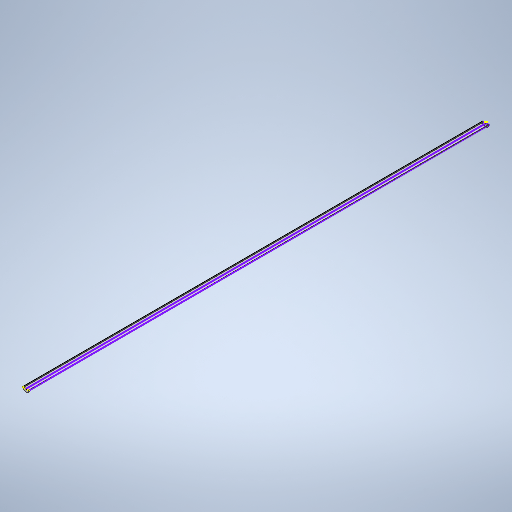
# Autodesk Inventor part: Tubo
Saved by Autodesk Inventor 2025.3 (Build 293356000, 356)
## iProperties
Created: 2025-11-02
Part Number: Tubo
Material: Genérico
Document SubType Name: Modeling
Designer: PAVILION
Density: 1 g/cm^3
Appearance: Valor por defecto
Author: PAVILION
Autodesk Inventor part; units mm, degrees
ref_plane "YZ Plane" through (0, 0, 0) normal (1, 0, 0) x (0, 1, 0)
ref_plane "XZ Plane" through (0, 0, 0) normal (0, 1, 0) x (-1, 0, 0)
ref_plane "XY Plane" through (0, 0, 0) normal (0, 0, 1) x (1, 0, 0)
sketch "Boceto1" plane through (0, 0, 0) normal (0, 0, 1) x (1, 0, 0)
  circle A0 centre (0, 0) radius 38.1
  circle A1 centre (0, 0) radius 34
  dimension "d0" = 76.2
  dimension "d1" = 68
  constraints: 2 centre point, 2 coincident
  measures "d0" diameter of A0
  measures "d1" diameter of A1
extrude "Extrusión1" add sketch "Boceto1" along normal blind 6100
sketch "Boceto2" plane through (0, 0, 6100) normal (0, 0, 1) x (1, 0, 0)
  circle A0 centre (0, 0) radius 39.5
  circle A1 centre (0, 0) radius 34 projected
  dimension "d4" = 79
  constraints: 1 centre point, 1 coincident
  measures "d4" diameter of A0
extrude "Extrusión2" add sketch "Boceto2" along normal blind 5 and the other way blind 5 contours A0 | A1
sketch "Boceto3" plane through (0, 0, 0) normal (0, 0, -1) x (-1, 0, 0)
  circle A0 centre (0, 0) radius 34 projected
  circle A1 centre (0, 0) radius 38.1 projected
  circle A2 centre (0, 0) radius 39.5 projected
extrude "Extrusión3" add sketch "Boceto3" along normal blind 5 and the other way blind 5 contours A0 | A1 | A2
sketch "Boceto4" plane through (0, 0, 0) normal (0, 1, 0) x (-1, 0, 0)
  line L0 (39.5, 6105) -> (-39.5, 6105) projected
  line L1 (39.5, 6105) -> (-39.5, 6105)
  line L2 (-39.5, 6105) -> (-39.5, -4.8433)
  line L3 (-39.5, -4.8433) -> (39.5, -4.8433)
  line L4 (39.5, -4.8433) -> (39.5, 6105)
  line L5 (0, 6105) -> (0, -4.8433)
  point P0 (0, 0)
  constraints: 10 end point, 2 midpoint, 2 parallel, 1 horizontal, 1 perpendicular
